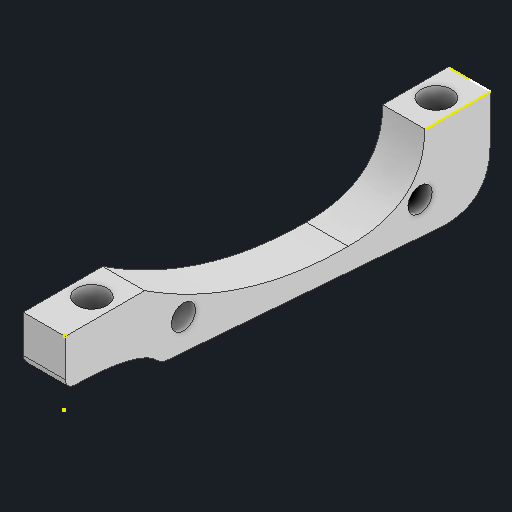
# Autodesk Inventor part: Pieza1
Saved by Autodesk Inventor 2024 (Build 280153000, 153)
## iProperties
Created: 2022-12-06
Part Number: Pieza1
Material: Genérico
Document SubType Name: Modeling
Designer: juanj
Density: 1 g/cm^3
Appearance: Valor por defecto
Author: juanj
Autodesk Inventor part; units mm, degrees
ref_plane "YZ Plane" through (0, 0, 0) normal (1, 0, 0) x (0, 1, 0)
ref_plane "XZ Plane" through (0, 0, 0) normal (0, 1, 0) x (-1, 0, 0)
ref_plane "XY Plane" through (0, 0, 0) normal (0, 0, 1) x (1, 0, 0)
sketch "Boceto3" plane through (0, 0, 0) normal (1, 0, 0) x (0, 1, 0)
  line L0 (0, -90) -> (0, -91)
  line L1 (0, -91) -> (10, -91)
  line L2 (10, -91) -> (10, -77)
  line L3 (-3.586, -60.6037) -> (-3.586, -77) construction
  line L4 (-3.586, -77) -> (10, -77) construction
  spline S0 degree 2 poles (-3.586, -60.6037) (-3.586, -77) (10, -77) knots 1 1 1 2 2 2
  line L5 (0, 0) -> (10, 0)
  line L6 (10, 0) -> (10, -17)
  line L7 (10, -17) -> (-3.586, -37.9742) construction
  line L8 (-3.586, -37.9742) -> (-3.586, -60.6037) construction
  spline S1 degree 2 poles (10, -17) (-3.586, -37.9742) (-3.586, -60.6037) knots 1 1 1 2 2 2
  line L9 (0, -91) -> (-10, -91) construction
  line L10 (-10, -91) -> (-10, -81) construction
  spline S2 degree 2 poles (0, -91) (-10, -91) (-10, -81) knots 1 1 1 2 2 2
  line L11 (-3.586, -76) -> (-2.6, -76)
  circle A0 centre (-2.6, -76) radius 2.6
  circle A1 centre (0.9686, -25.3255) radius 2.6
  line L12 (0, 0) -> (0, -17) construction
  line L13 (0, -17) -> (-5.2, -20.5234) construction
  spline S3 degree 2 poles (0, 0) (0, -17) (-5.2, -20.5234) knots 1 1 1 2 2 2
  line L14 (-5.2, -20.5234) -> (-10, -81)
  dimension "d36" = 1
  dimension "d40" = 10
  dimension "d41" = 17
  constraints: 14 end point, 2 centre point, 2 perpendicular, 2 vertical, 1 coincident, 1 horizontal, 1 point on line, 12 other
  measures "d36" distance of L0.start L0.end
  measures "d40" distance of L5.start L5.end
  measures "d41" distance of L5.end L6.end
extrude "Extrusión4" add sketch "Boceto3" against normal blind 9
fillet "Empalme1" radius 2 1 edges at (-4.5, -5.2, -20.5234)
fillet "Empalme2" radius 2 1 edges at (-4.5, 0, 0)
sketch "Boceto4" plane through (0, 10, -77) normal (0, 1, 0) x (1, 0, 0)
  line L0 (0, 14) -> (0, 0) projected
  line L1 (0, 14) -> (-4.5, 14)
  line L2 (0, 14) -> (-9, 14) projected
  point P0 (0, -77)
  constraints: 2 end point, 1 midpoint
sketch "Boceto5" plane through (0, 10, 0) normal (0, 1, 0) x (1, 0, 0)
  point P0 (0, 0)
sketch "Boceto7" plane through (0, 10, -77) normal (0, 1, 0) x (1, 0, 0)
  line L0 (0, 14) -> (-9, 14) projected
  line L1 (-4.5, 14) -> (-4.5, 7)
  circle A0 centre (-4.5, 7) radius 3.25
  line L2 (-4.5, 7) -> (-4.5, -66.8)
  circle A1 centre (-4.5, -66.8) radius 3.25
  point P0 (0, -77)
  dimension "d67" = 7
  dimension "d68" = 6.5
  dimension "d69" = 73.8
  dimension "d70" = 6.5
  constraints: 4 end point, 2 centre point, 2 coincident, 2 vertical, 1 midpoint
  measures "d67" distance of L1.start L1.end
  measures "d68" diameter of A0
  measures "d69" distance of L2.start L2.end
  measures "d70" diameter of A1
extrude "Extrusión7" cut sketch "Boceto7" against normal blind 20
sketch "Boceto8" plane through (-9, -10, -81) normal (0, -0.9969, 0.0791) x (1, 0, 0)
  point P0 (9, 81.5373)
sketch "Boceto9" plane through (0, 10, 0) normal (0, 1, 0) x (1, 0, 0)
  point P0 (0, 0)
